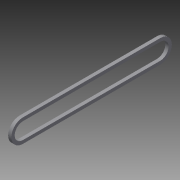
# Autodesk Inventor part: chain
Saved by Autodesk Inventor 2015 SP1 (Build 190203100, 203)
## iProperties
Created: 2014-12-23
Part Number: chain
Material: Generic
Document SubType Name: Modeling
Designer: Jarod
Density: 1 g/cm^3
Appearance: Default
Author: Jarod
Autodesk Inventor part; units mm, degrees
ref_plane "YZ Plane" through (0, 0, 0) normal (1, 0, 0) x (0, 1, 0)
ref_plane "XZ Plane" through (0, 0, 0) normal (0, 1, 0) x (-1, 0, 0)
ref_plane "XY Plane" through (0, 0, 0) normal (0, 0, 1) x (1, 0, 0)
sketch "Sketch1" plane through (0, 0, 0) normal (1, 0, 0) x (0, 1, 0)
  line L0 (0, 0) -> (0, -266.7) construction
  line L1 (0, 0) -> (15.875, 0) construction
  line L2 (0, 0) -> (-15.875, 0) construction
  line L3 (0, -266.7) -> (15.875, -266.7) construction
  line L4 (0, -266.7) -> (15.875, -266.7) construction
  line L5 (0, -266.7) -> (-15.875, -266.7) construction
  line L6 (0, -266.7) -> (15.875, -266.7) construction
  arc A0 (15.875, 0) -> (-15.875, 0) centre (0, 0) ccw
  line L7 (15.875, 0) -> (15.875, -266.7)
  line L8 (-15.875, 0) -> (-15.875, -266.7)
  arc A1 (-15.875, -266.7) -> (15.875, -266.7) centre (0, -266.7) ccw
  line L9 (22.225, -266.7) -> (22.225, 0)
  arc A2 (22.225, 0) -> (-22.225, 0) centre (0, 0) ccw
  line L10 (-22.225, 0) -> (-22.225, -266.7)
  arc A3 (-22.225, -266.7) -> (22.225, -266.7) centre (0, -266.7) ccw
  dimension "d0" = 266.7
  dimension "d3" = 15.875
  dimension "d4" = 15.875
  dimension "d5" = 15.875
  dimension "d6" = 0
  dimension "d7" = 15.875
  dimension "d8" = 180
  dimension "d9" = 15.875
  dimension "d10" = 15.875
  dimension "d11" = 6.35
  constraints: 22 end point, 8 point on circle, 6 horizontal, 4 centre point, 2 collinear, 1 coincident, 1 vertical, 3 other
  measures "d0" distance of L0.start L0.end
  measures "d3" distance of L1.start L1.end
  measures "d4" distance of L1.start L2.end
  measures "d5" distance of L0.end L3.end
  measures "d6" distance between parallel lines of L3 L4
  measures "d7" distance of L0.end L5.end
  measures "d8" angle of L5 L6
  measures "d9" radius of A0
  measures "d10" radius of A1
  measures "d11" distance between parallel lines of L9 L7
extrude "Extrusion1" add sketch "Sketch1" along normal blind 6.35
body "Solid1"
